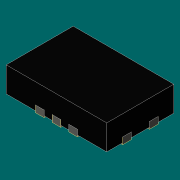
# Autodesk Inventor part: udb10LeadQFN3x2
Saved by Autodesk Inventor 2016 (Build 200138000, 138)
## iProperties
Created: 2016-02-09
Part Number: udb10LeadQFN3x2
Material: ABS Plastic
Document SubType Name: Modeling
Designer: Sawaiz
Density: 1.06 g/cm^3
Appearance: Smooth - Black
Author: Sawaiz
Autodesk Inventor part; units mm, degrees
ref_plane "YZ Plane" through (0, 0, 0) normal (1, 0, 0) x (0, 1, 0)
ref_plane "XZ Plane" through (0, 0, 0) normal (0, 1, 0) x (-1, 0, 0)
ref_plane "XY Plane" through (0, 0, 0) normal (0, 0, 1) x (1, 0, 0)
sketch "Sketch1" plane through (0, 0, 0) normal (0, 0, 1) x (1, 0, 0)
  line L0 (-1, -1.5) -> (1, -1.5)
  line L1 (1, -1.5) -> (1, 1.5)
  line L2 (1, 1.5) -> (-1, 1.5)
  line L3 (-1, 1.5) -> (-1, -1.5)
  line L4 (-1, -1.5) -> (1, 1.5) construction
  line L5 (1, -1.5) -> (-1, 1.5) construction
  point P0 (0, 0)
  dimension "d0" = 2
  dimension "d1" = 3
  constraints: 12 end point, 2 midpoint, 2 parallel, 1 horizontal, 1 perpendicular
  measures "d0" distance of L2.end L1.end
  measures "d1" distance of L1.end L0.end
extrude "Extrusion1" add sketch "Sketch1" along normal blind 0.75
sketch "Sketch2" plane through (0, 0, 0) normal (0, 0, -1) x (-1, 0, 0)
  line L0 (1, -1.5) -> (-1, -1.5) projected
  line L1 (1, 1.5) -> (1, -1.5) projected
  line L2 (-1, 1.5) -> (1, 1.5) projected
  line L3 (-1, -1.5) -> (-1, 1.5) projected
  line L4 (-1, -1.5) -> (-1, 1.5) projected
  line L5 (-1, -0.13) -> (-0.73, -0.13)
  line L6 (-0.73, 0.13) -> (-1, 0.13)
  line L7 (-1, 0.13) -> (-1, -0.13)
  arc A0 (-0.73, -0.13) -> (-0.73, 0.13) centre (-0.73, 0) ccw
  point P0 (0, 0)
  point P1 (-1, 0)
  dimension "d4" = 0.13
  dimension "d5" = 0.27
  constraints: 6 end point, 2 midpoint, 2 point on circle, 2 tangent, 1 centre point, 1 horizontal, 1 parallel, 1 point on line
  measures "d4" radius of A0
  measures "d5" distance from line of L3 A0.centre
extrude "Extrusion2" cut sketch "Sketch2" against normal blind 0.15 contours L3 L6 A0 L5
pattern_linear "Rectangular Pattern1" count 3 spacing 0.5 along (0, 1, 0) of "Extrusion2" first direction both ways yes
sketch "Sketch3" plane through (0, 0, 0) normal (0, 0, -1) x (-1, 0, 0)
  line L0 (1, 1.5) -> (1, -1.5) projected
  line L1 (-1, 1.5) -> (1, 1.5) projected
  line L2 (-1, 0.63) -> (-1, 1.5) projected
  line L3 (-1, 0.63) -> (-0.73, 0.63) projected
  arc A0 (-0.73, 0.37) -> (-0.73, 0.63) centre (-0.73, 0.5) ccw projected
  line L4 (-0.73, 0.37) -> (-1, 0.37) projected
  line L5 (-1, 0.13) -> (-1, 0.37) projected
  line L6 (-1, 0.13) -> (-0.73, 0.13) projected
  arc A1 (-0.73, -0.13) -> (-0.73, 0.13) centre (-0.73, 0) ccw projected
  line L7 (-0.73, -0.13) -> (-1, -0.13) projected
  line L8 (-1, -0.37) -> (-1, -0.13) projected
  line L9 (-1, -0.37) -> (-0.73, -0.37) projected
  arc A2 (-0.73, -0.63) -> (-0.73, -0.37) centre (-0.73, -0.5) ccw projected
  line L10 (-0.73, -0.63) -> (-1, -0.63) projected
  line L11 (-1, -1.5) -> (-1, -0.63) projected
  line L12 (1, -1.5) -> (-1, -1.5) projected
  line L13 (-0.53, 1.5) -> (-0.27, 1.5)
  line L14 (-0.27, 1.5) -> (-0.27, 1.03)
  line L15 (-0.53, 1.03) -> (-0.53, 1.5)
  arc A3 (-0.53, 1.03) -> (-0.27, 1.03) centre (-0.4, 1.03) ccw
  line L16 (-1, 1.5) -> (1, 1.5) projected
  point P0 (0, 0)
  point P1 (-0.4, 1.5)
  point P2 (0, 1.5)
  dimension "d11" = 0.13
  dimension "d12" = 0.4
  dimension "d13" = 0.47
  constraints: 6 end point, 2 midpoint, 2 point on circle, 2 tangent, 1 centre point, 1 horizontal, 1 parallel, 1 perpendicular, 1 point on line
  measures "d11" radius of A3
  measures "d12" distance of point (-0.4, 1.5) point (0, 1.5)
  measures "d13" distance from line of L1 A3.centre
extrude "Extrusion3" cut sketch "Sketch3" against normal blind 0.15 contours L14 A3 L15 L1
mirror "Mirror2" about plane through (0, 0, 0) normal (1, 0, 0) of "Extrusion3"
mirror "Mirror3" about plane through (0, 0, 0) normal (0, 1, 0) of "Extrusion3", "Mirror2"
sketch "Sketch4" plane through (0, 0, 0) normal (0, 0, -1) x (-1, 0, 0)
  line L0 (0.53, -1.03) -> (0.53, -1.5) projected
  line L1 (1, -1.5) -> (0.53, -1.5) projected
  line L2 (1, 1.5) -> (1, -1.5) projected
  line L3 (0.53, 1.5) -> (1, 1.5) projected
  line L4 (0.53, 1.5) -> (0.53, 1.03) projected
  arc A0 (0.27, 1.03) -> (0.53, 1.03) centre (0.4, 1.03) ccw projected
  line L5 (0.27, 1.03) -> (0.27, 1.5) projected
  line L6 (-0.27, 1.5) -> (0.27, 1.5) projected
  line L7 (-0.27, 1.5) -> (-0.27, 1.03) projected
  arc A1 (-0.53, 1.03) -> (-0.27, 1.03) centre (-0.4, 1.03) ccw projected
  line L8 (-0.53, 1.03) -> (-0.53, 1.5) projected
  line L9 (-1, 1.5) -> (-0.53, 1.5) projected
  line L10 (-1, 0.63) -> (-1, 1.5) projected
  line L11 (-1, 0.63) -> (-0.73, 0.63) projected
  arc A2 (-0.73, 0.37) -> (-0.73, 0.63) centre (-0.73, 0.5) ccw projected
  line L12 (-0.73, 0.37) -> (-1, 0.37) projected
  line L13 (-1, 0.13) -> (-1, 0.37) projected
  line L14 (-1, 0.13) -> (-0.73, 0.13) projected
  arc A3 (-0.73, -0.13) -> (-0.73, 0.13) centre (-0.73, 0) ccw projected
  line L15 (-0.73, -0.13) -> (-1, -0.13) projected
  line L16 (-1, -0.37) -> (-1, -0.13) projected
  line L17 (-1, -0.37) -> (-0.73, -0.37) projected
  arc A4 (-0.73, -0.63) -> (-0.73, -0.37) centre (-0.73, -0.5) ccw projected
  line L18 (-0.73, -0.63) -> (-1, -0.63) projected
  line L19 (-1, -1.5) -> (-1, -0.63) projected
  line L20 (-0.53, -1.5) -> (-1, -1.5) projected
  line L21 (-0.53, -1.5) -> (-0.53, -1.03) projected
  arc A5 (-0.27, -1.03) -> (-0.53, -1.03) centre (-0.4, -1.03) ccw projected
  line L22 (-0.27, -1.03) -> (-0.27, -1.5) projected
  line L23 (0.27, -1.5) -> (-0.27, -1.5) projected
  line L24 (0.27, -1.5) -> (0.27, -1.03) projected
  arc A6 (0.53, -1.03) -> (0.27, -1.03) centre (0.4, -1.03) ccw projected
  line L25 (-0.27, 1.5) -> (-0.27, 1.03) projected
  line L26 (-0.27, 1.5) -> (-0.53, 1.5)
  line L27 (-0.53, 1.5) -> (-0.53, 0.8)
  line L28 (-0.53, 0.8) -> (-0.27, 0.8)
  line L29 (-0.27, 0.8) -> (-0.27, 1.5)
  line L30 (-0.53, 1.03) -> (-0.53, 1.5) projected
  point P0 (0, 0)
  dimension "d16" = 0.7
  constraints: 8 end point, 2 parallel, 1 collinear, 1 horizontal, 1 perpendicular
  measures "d16" distance between parallel lines of L26 L28
extrude "Extrusion4" cut sketch "Sketch4" against normal blind 0.15 contours L7 A1 L8 L26 | L29 L28 L27 A1
sketch "Sketch6" plane through (0, 0, 0) normal (0, 0, -1) x (-1, 0, 0)
  line L0 (-0.15, -0.45) -> (0.1, -0.45)
  line L1 (0.1, -0.45) -> (0.1, 0.45)
  line L2 (0.1, 0.45) -> (-0.15, 0.45)
  line L3 (-0.15, 0.45) -> (-0.15, -0.45)
  line L4 (-0.15, -0.45) -> (0.1, 0.45) construction
  line L5 (0.1, -0.45) -> (-0.15, 0.45) construction
  line L6 (0, 0) -> (-0.025, 0) construction
  dimension "d22" = 0.1
  dimension "d23" = 0.25
  dimension "d24" = 0.9
  constraints: 14 end point, 2 horizontal, 2 midpoint, 2 parallel, 1 perpendicular
  measures "d22" distance from line of L1 L6.start
  measures "d23" distance of L0.start L0.end
  measures "d24" distance between parallel lines of L2 L0
sketch "Sketch7" plane through (0, 0, 0) normal (0, 0, -1) x (-1, 0, 0)
  line L0 (-0.53, 0.8) -> (-0.53, 1.5) projected
  line L1 (-1, 1.5) -> (-0.53, 1.5) projected
  line L2 (-1, 0.63) -> (-1, 1.5) projected
  line L3 (-1, 0.63) -> (-0.73, 0.63) projected
  arc A0 (-0.73, 0.37) -> (-0.73, 0.63) centre (-0.73, 0.5) ccw projected
  line L4 (-0.73, 0.37) -> (-1, 0.37) projected
  line L5 (-1, 0.13) -> (-1, 0.37) projected
  line L6 (-1, 0.13) -> (-0.73, 0.13) projected
  arc A1 (-0.73, -0.13) -> (-0.73, 0.13) centre (-0.73, 0) ccw projected
  line L7 (-0.73, -0.13) -> (-1, -0.13) projected
  line L8 (-1, -0.37) -> (-1, -0.13) projected
  line L9 (-1, -0.37) -> (-0.73, -0.37) projected
  arc A2 (-0.73, -0.63) -> (-0.73, -0.37) centre (-0.73, -0.5) ccw projected
  line L10 (-0.73, -0.63) -> (-1, -0.63) projected
  line L11 (-1, -1.5) -> (-1, -0.63) projected
  line L12 (-0.53, -1.5) -> (-1, -1.5) projected
  line L13 (-0.53, -1.5) -> (-0.53, -1.03) projected
  arc A3 (-0.27, -1.03) -> (-0.53, -1.03) centre (-0.4, -1.03) ccw projected
  line L14 (-0.27, -1.03) -> (-0.27, -1.5) projected
  line L15 (0.27, -1.5) -> (-0.27, -1.5) projected
  line L16 (0.27, -1.5) -> (0.27, -1.03) projected
  arc A4 (0.53, -1.03) -> (0.27, -1.03) centre (0.4, -1.03) ccw projected
  line L17 (0.53, -1.03) -> (0.53, -1.5) projected
  line L18 (1, -1.5) -> (0.53, -1.5) projected
  line L19 (1, 1.5) -> (1, -1.5) projected
  line L20 (0.53, 1.5) -> (1, 1.5) projected
  line L21 (0.53, 1.5) -> (0.53, 1.03) projected
  arc A5 (0.27, 1.03) -> (0.53, 1.03) centre (0.4, 1.03) ccw projected
  line L22 (0.27, 1.03) -> (0.27, 1.5) projected
  line L23 (-0.27, 1.5) -> (0.27, 1.5) projected
  line L24 (-0.27, 1.5) -> (-0.27, 0.8) projected
  line L25 (-0.27, 0.8) -> (-0.53, 0.8) projected
  line L26 (1, -0.13) -> (0.63, -0.13)
  line L27 (0.63, 0.13) -> (1, 0.13)
  line L28 (1, 0.13) -> (1, -0.13)
  arc A6 (0.63, 0.13) -> (0.63, -0.13) centre (0.63, 0) ccw
  point P0 (0, 0)
  point P1 (1, 0)
  dimension "d25" = 0.13
  dimension "d26" = 0.37
  constraints: 6 end point, 2 midpoint, 2 point on circle, 2 tangent, 1 centre point, 1 horizontal, 1 parallel, 1 point on line
  measures "d25" radius of A6
  measures "d26" distance from line of L19 A6.centre
extrude "Extrusion6" cut sketch "Sketch7" against normal blind 0.15 contours L19 L26 A6 L27
pattern_linear "Rectangular Pattern2" count 3 spacing 0.5 along (0, -1, 0) of "Extrusion6" first direction both ways yes
extrude "Extrusion7" cut sketch "Sketch6" against normal blind 0.15
sketch "Sketch8" plane through (0, 0, 0) normal (0, 0, -1) x (-1, 0, 0)
  line L0 (0.1, -0.45) -> (-0.15, -0.45) projected
  line L1 (0.1, 0.45) -> (0.1, -0.45) projected
  line L2 (-0.15, 0.45) -> (0.1, 0.45) projected
  line L3 (-0.15, -0.45) -> (-0.15, 0.45) projected
  line L4 (0.1, 0.45) -> (0.1, -0.45) projected
  line L5 (0.1, 0.45) -> (-0.15, -0.45) construction
  circle A0 centre (-0.025, 0) radius 0.5
  point P0 (0, 0)
  dimension "d34" = 1
  constraints: 2 end point, 1 centre point, 1 coincident, 1 midpoint
  measures "d34" diameter of A0
extrude "Extrusion8" cut sketch "Sketch8" against normal blind 0.01
sketch "Sketch9" plane through (0, 0, 0) normal (0, 0, -1) x (-1, 0, 0)
  line L0 (-0.53, 0.8) -> (-0.53, 1.5) projected
  line L1 (-0.27, 0.8) -> (-0.53, 0.8) projected
  line L2 (-0.27, 1.5) -> (-0.27, 0.8) projected
  line L3 (-0.53, 1.5) -> (-0.27, 1.5) projected
  line L4 (0.53, 1.03) -> (0.53, 1.5) projected
  line L5 (0.27, 1.5) -> (0.53, 1.5) projected
  line L6 (0.27, 1.5) -> (0.27, 1.03) projected
  arc A0 (0.27, 1.03) -> (0.53, 1.03) centre (0.4, 1.03) ccw projected
  line L7 (1, 0.63) -> (1, 0.37) projected
  line L8 (0.63, 0.63) -> (1, 0.63) projected
  arc A1 (0.63, 0.63) -> (0.63, 0.37) centre (0.63, 0.5) ccw projected
  line L9 (1, 0.37) -> (0.63, 0.37) projected
  line L10 (1, 0.13) -> (1, -0.13) projected
  line L11 (0.63, 0.13) -> (1, 0.13) projected
  arc A2 (0.63, 0.13) -> (0.63, -0.13) centre (0.63, 0) ccw projected
  line L12 (1, -0.13) -> (0.63, -0.13) projected
  line L13 (1, -0.37) -> (1, -0.63) projected
  line L14 (0.63, -0.37) -> (1, -0.37) projected
  arc A3 (0.63, -0.37) -> (0.63, -0.63) centre (0.63, -0.5) ccw projected
  line L15 (1, -0.63) -> (0.63, -0.63) projected
  line L16 (0.53, -1.03) -> (0.53, -1.5) projected
  arc A4 (0.53, -1.03) -> (0.27, -1.03) centre (0.4, -1.03) ccw projected
  line L17 (0.27, -1.5) -> (0.27, -1.03) projected
  line L18 (0.53, -1.5) -> (0.27, -1.5) projected
  line L19 (-0.53, -1.03) -> (-0.53, -1.5) projected
  line L20 (-0.27, -1.5) -> (-0.53, -1.5) projected
  line L21 (-0.27, -1.5) -> (-0.27, -1.03) projected
  arc A5 (-0.27, -1.03) -> (-0.53, -1.03) centre (-0.4, -1.03) ccw projected
  line L22 (0.1, -0.45) -> (-0.15, -0.45) projected
  line L23 (0.1, 0.45) -> (0.1, -0.45) projected
  line L24 (-0.15, 0.45) -> (0.1, 0.45) projected
  line L25 (-0.15, -0.45) -> (-0.15, 0.45) projected
  line L26 (-0.73, -0.63) -> (-1, -0.63) projected
  arc A6 (-0.73, -0.63) -> (-0.73, -0.37) centre (-0.73, -0.5) ccw projected
  line L27 (-1, -0.37) -> (-0.73, -0.37) projected
  line L28 (-1, -0.63) -> (-1, -0.37) projected
  line L29 (-0.73, -0.13) -> (-1, -0.13) projected
  arc A7 (-0.73, -0.13) -> (-0.73, 0.13) centre (-0.73, 0) ccw projected
  line L30 (-1, 0.13) -> (-0.73, 0.13) projected
  line L31 (-1, -0.13) -> (-1, 0.13) projected
  line L32 (-0.73, 0.37) -> (-1, 0.37) projected
  arc A8 (-0.73, 0.37) -> (-0.73, 0.63) centre (-0.73, 0.5) ccw projected
  line L33 (-1, 0.63) -> (-0.73, 0.63) projected
  line L34 (-1, 0.37) -> (-1, 0.63) projected
  point P0 (0, 0)
extrude "Extrusion9" add sketch "Sketch9" against normal blind 0.15 and the other way blind 0.05 separate body
body "Solid1"
body "Solid2"
